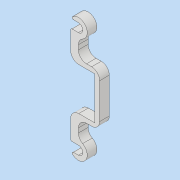
# Autodesk Inventor part: batteryConnectorHolder
Saved by Autodesk Inventor 2017 (Build 210142000, 142)
## iProperties
Created: 2019-07-14
Part Number: batteryConnectorHolder
Material: ABS Plastic
Document SubType Name: Modeling
Designer: techn
Density: 1.06 g/cm^3
Appearance: Smooth - White
Author: techn
Autodesk Inventor part; units mm, degrees
ref_plane "YZ Plane" through (0, 0, 0) normal (1, 0, 0) x (0, 1, 0)
ref_plane "XZ Plane" through (0, 0, 0) normal (0, 1, 0) x (-1, 0, 0)
ref_plane "XY Plane" through (0, 0, 0) normal (0, 0, 1) x (1, 0, 0)
sketch "Sketch1" plane through (0, 0, 0) normal (0, 0, 1) x (1, 0, 0)
  arc A0 (0, -1.7145) -> (0, 1.7145) centre (0, 0) ccw
  arc A1 (-3.0427, -1.7145) -> (0, 3.4925) centre (0, 0) ccw
  arc A2 (0, 40.1955) -> (0, 43.6245) centre (0, 41.91) ccw
  arc A3 (0, 38.4175) -> (-3.0427, 43.6245) centre (0, 41.91) ccw
  line L0 (0, 40.1955) -> (-3.0427, 40.1955)
  line L1 (-3.0427, 1.7145) -> (0, 1.7145)
  line L2 (-3.0427, 29.337) -> (6.4823, 29.337)
  line L3 (6.4823, 29.337) -> (6.4823, 12.573)
  line L4 (6.4823, 12.573) -> (-3.0427, 12.573)
  line L5 (0, 3.4925) -> (0, 10.795)
  line L6 (0, 10.795) -> (8.3873, 10.795)
  line L7 (8.3873, 10.795) -> (8.3873, 31.115)
  line L8 (8.3873, 31.115) -> (0, 31.115)
  line L9 (0, 31.115) -> (0, 38.4175)
  line L10 (0, 43.6245) -> (-3.0427, 43.6245)
  line L11 (0, -1.7145) -> (-3.0427, -1.7145)
  line L12 (-3.0427, 40.1955) -> (-3.0427, 29.337)
  line L13 (-3.0427, 12.573) -> (-3.0427, 1.7145)
  point P0 (8.3873, 20.955)
  point P1 (6.4823, 20.955)
  dimension "d0" = 3.429
  dimension "d1" = 6.985
  dimension "d2" = 41.91
  dimension "d5" = 20.955
  dimension "d6" = 16.764
  dimension "d7" = 9.525
  dimension "d8" = 20.32
  dimension "d9" = 11.43
  constraints: 28 end point, 8 point on circle, 6 perpendicular, 4 centre point, 4 horizontal, 3 coincident, 3 tangent, 3 vertical alignment, 2 equal radius, 2 midpoint, 2 parallel, 2 point on line, 1 horizontal alignment, 1 vertical
  measures "d0" diameter of A0
  measures "d1" diameter of A1
  measures "d2" distance of point (0, 0) A2.centre
  measures "d5" vertical distance of point (0, 0) point (8.387, 20.955)
  measures "d6" distance of L2.end L3.end
  measures "d7" distance of L2.start L2.end
  measures "d8" distance of L6.end L7.end
  measures "d9" distance between parallel lines of L7 L12
extrude "Extrusion1" add sketch "Sketch1" along normal blind 3.81
fillet "Fillet1" radius 3.175 8 edges at (0, 31.115, 1.905) (8.3873, 31.115, 1.905) (8.3873, 10.795, 1.905) (0, 10.795, 1.905) (-3.0427, 12.573, 1.905) (-3.0427, 29.337, 1.905) (0, 3.4925, 1.905) (0, 38.4175, 1.905)
fillet "Fillet2" radius 0.508 4 edges at (-3.0427, -1.7145, 1.905) (-3.0427, 1.7145, 1.905) (-3.0427, 40.1955, 1.905) (-3.0427, 43.6245, 1.905)
equation "\"d5\" = 0.5 * d2"
body "Solid1"
